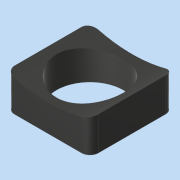
# Autodesk Inventor part: CoilHolder
Saved by Autodesk Inventor 2017 (Build 210142000, 142)
## iProperties
Created: 2017-11-03
Part Number: CoilHolder
Material: ABS Plastic
Document SubType Name: Modeling
Designer: Derek Wider
Density: 1.06 g/cm^3
Appearance: Smooth - Black
Author: Derek Wider
Autodesk Inventor part; units mm, degrees
ref_plane "YZ Plane" through (0, 0, 0) normal (1, 0, 0) x (0, 1, 0)
ref_plane "XZ Plane" through (0, 0, 0) normal (0, 1, 0) x (-1, 0, 0)
ref_plane "XY Plane" through (0, 0, 0) normal (0, 0, 1) x (1, 0, 0)
sketch "Sketch1" plane through (0, 0, 0) normal (0, 0, 1) x (1, 0, 0)
  line L0 (0, 0) -> (31.75, 0)
  arc A0 (0, 12.7) -> (31.75, 12.7) centre (15.875, 60.9558) ccw
  line L1 (0, 12.7) -> (0, 0)
  line L2 (31.75, 12.7) -> (31.75, 0)
  dimension "d0" = 50.8
  dimension "d1" = 31.75
  dimension "d2" = 12.7
  constraints: 6 end point, 2 point on circle, 1 centre point, 1 horizontal, 1 horizontal alignment, 1 parallel, 1 vertical
  measures "d0" radius of A0
  measures "d1" distance of L0.start L0.end
  measures "d2" distance of L2.start L0.end
extrude "Extrusion1" add sketch "Sketch1" along normal blind 31.75
sketch "Sketch2" plane through (0, 0, 0) normal (0, -1, 0) x (1, 0, 0)
  line L0 (31.75, 0) -> (31.75, 31.75) projected
  circle A0 centre (15.875, 15.875) radius 12.7
  line L1 (0, 0) -> (31.75, 0) projected
  line L2 (15.875, 15.875) -> (0, 15.875) construction
  line L3 (0, 0) -> (0, 31.75) construction
  line L4 (15.875, 15.875) -> (31.75, 15.875) construction
  line L5 (15.875, 15.875) -> (15.875, 31.75) construction
  line L6 (15.875, 15.875) -> (15.875, 0) construction
  line L7 (0, 31.75) -> (31.75, 31.75) construction
  dimension "d5" = 25.4
  constraints: 8 end point, 4 midpoint, 2 collinear, 1 centre point, 1 perpendicular, 1 vertical
  measures "d5" diameter of A0
extrude "Extrusion2" cut sketch "Sketch2" against normal through all
fillet "Fillet1" radius 3.175 4 edges at (31.75, 6.35, 31.75) (0, 6.35, 31.75) (31.75, 6.35, 0) (0, 6.35, 0)
body "Solid1"
